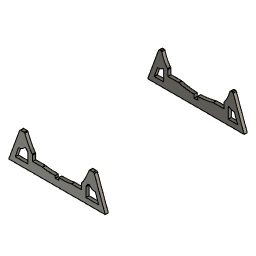
Revell Flower Class stand (Autodesk Fusion 360 design; units mm, degrees)
Autodesk Fusion 360 part; units mm, degrees
note: some values were not read from the file. Chosen so that the rebuilt part matches the saved one: which face or edge a step refers to.
ref_plane "WorkPlane1" through (0, -135, 0) normal (0, 1, 0) x (0, 0, 1) in component "Fore"
sketch "Sketch1" plane through (0, -135, 0) normal (0, 1, 0) x (1, 0, 0) in component "Fore"
  line L0 (0, 0) -> (0, -12.5)
  line L1 (0, -12.5) -> (-3.5, -12.5)
  line L2 (-3.5, -12.5) -> (-3.5, -17)
  spline S0 degree 5 poles (-3.5, -17) (-4.4939, -17) (-6.4799, -17.0057) (-9.4532, -17.0312) (-13.4085, -17.1077) (-18.3463, -17.343) (-22.2994, -17.7362) (-25.2695, -18.2105) (-27.2527, -18.6198) (-28.245, -18.8477) knots 0 0 0 0 0 0 0.2 0.4 0.6 0.8 1 1 1 1 1 1
  line L3 (-28.245, -18.8477) -> (-47.4725, -18.8477)
  line L4 (-47.4725, -18.8477) -> (-47.4725, -30.1587)
  spline S1 degree 5 poles (-47.4725, -30.1587) (-47.8872, -30.6443) (-48.7402, -31.6972) (-50.0906, -33.5222) (-52.0431, -36.4804) (-54.8605, -41.4812) (-57.606, -47.1812) (-60.0804, -52.8922) (-61.9442, -57.4399) (-62.9296, -59.899) knots 0 0 0 0 0 0 0.2 0.4 0.6 0.8 1 1 1 1 1 1
  line L5 (-62.9296, -59.899) -> (-72.0582, -59.899)
  line L6 (-72.0582, -59.899) -> (-93.742, 0)
  line L7 (-93.742, 0) -> (0, 0)
  line L8 (-60.4227, -53.6433) -> (-65.4365, -66.1546)
  line L9 (-0.969, -17) -> (-6.031, -17)
  line L10 (-25.7289, -18.2698) -> (-30.7611, -19.4256)
  line L11 (-74.7277, -28.7021) -> (-81.0107, -10.108)
  line L12 (-81.0107, -10.108) -> (-56.4844, -10.108)
  line L13 (-56.4844, -10.108) -> (-56.4844, -29.2553)
  line L14 (-56.4844, -29.2553) -> (-59.3576, -33.4494)
  spline S2 degree 5 poles (-59.3576, -33.4494) (-59.567, -33.755) (-60.0141, -34.2929) (-60.7709, -34.8796) (-61.8493, -35.2265) (-62.983, -34.9858) (-63.6467, -34.1638) (-64.3685, -32.9555) (-65.6314, -31.5945) (-67.452, -30.2924) (-69.7221, -29.2481) (-71.72, -28.7519) (-73.231, -28.6255) (-74.2302, -28.6572) (-74.7277, -28.7021) knots 0 0 0 0 0 0 0.1 0.2 0.3 0.4 0.5 0.6 0.7 0.8 0.9 1 1 1 1 1 1
  line L15 (-72.7235, -28.5213) -> (-76.7319, -28.8828)
  line L16 (-62.8657, -35.095) -> (-64.2557, -33.3052)
  line L17 (-57.9122, -31.3395) -> (-60.8031, -35.5592)
  point P0 (-63.5607, -34.2001)
  dimension "d2" = 12.5
  dimension "d3" = 4.5
  dimension "d4" = 3.5
  constraint coincident L0.start L7.end
  constraint vertical L0
  constraint perpendicular L0 L1
  constraint perpendicular L1 L2
  constraint horizontal L3
  constraint perpendicular L3 L4
  constraint horizontal L5
  constraint perpendicular L0 L7
  constraint midpoint S1.end L8
  constraint midpoint L2.end L9
  constraint horizontal L9
  constraint midpoint S0.end L10
  constraint horizontal L12
  constraint perpendicular L12 L13
  constraint midpoint L11.start L15
  constraint midpoint P0 L16
  constraint midpoint L14.end L17
  measures "d2" distance of L0.start L0.end
  measures "d3" distance of L1.end L2.end
  measures "d4" distance of L0.end L1.end
ref_plane "WorkPlane1" through (0, 135, 0) normal (0, 1, 0) x (0, 0, 1) in component "Aft"
sketch "Sketch1 (2)" plane through (0, 135, 0) normal (0, 1, 0) x (1, 0, 0) in component "Aft"
  line L0 (0, 0) -> (0, -12.5)
  line L1 (0, -12.5) -> (-3.5, -12.5)
  line L2 (-3.5, -12.5) -> (-3.5, -19)
  spline S0 degree 5 poles (-3.5, -19) (-4.3766, -19) (-6.2365, -19.0347) (-9.3458, -19.191) (-14.0327, -19.5941) (-20.4233, -20.4205) (-25.6959, -21.3969) (-29.6354, -22.3657) (-32.2417, -23.1312) (-33.54, -23.5438) knots 0 0 0 0 0 0 0.2 0.4 0.6 0.8 1 1 1 1 1 1
  line L3 (-33.54, -23.5438) -> (-54.6225, -23.5438)
  line L4 (-54.6225, -23.5438) -> (-54.6225, -35.6286)
  spline S1 degree 5 poles (-54.6225, -35.6286) (-55.2677, -36.2626) (-56.496, -37.575) (-58.1518, -39.6766) (-60.0494, -42.7526) (-62.1582, -47.2156) (-63.8351, -51.5517) (-65.178, -55.4393) (-66.1249, -58.3579) (-66.6112, -59.899) knots 0 0 0 0 0 0 0.2 0.4 0.6 0.8 1 1 1 1 1 1
  line L5 (-72.0582, -59.899) -> (-93.742, 0)
  line L6 (-72.0582, -59.899) -> (-66.6112, -59.899)
  line L7 (-65.3783, -55.9921) -> (-67.8442, -63.8058)
  line L8 (-53.0217, -34.0557) -> (-56.2233, -37.2015)
  line L9 (-93.742, 0) -> (0, 0)
  line L10 (-74.5428, -28.526) -> (-81.0107, -10.108)
  line L11 (-81.0107, -10.108) -> (-62.7924, -10.108)
  line L12 (-62.7924, -10.108) -> (-62.7924, -32.6534)
  spline S2 degree 5 poles (-62.7924, -32.6534) (-63.1413, -32.3681) (-63.8532, -31.8115) (-64.9633, -31.0185) (-66.5337, -30.0508) (-68.7209, -29.0636) (-70.7629, -28.564) (-72.5414, -28.4344) (-73.8545, -28.4744) (-74.5428, -28.526) knots 0 0 0 0 0 0 0.2 0.4 0.6 0.8 1 1 1 1 1 1
  line L13 (-72.8582, -28.3997) -> (-76.2275, -28.6524)
  line L14 (-1.2608, -19) -> (-5.7392, -19)
  line L15 (-30.2257, -22.4904) -> (-36.8542, -24.5973)
  point P0 (-81.0107, -10.108)
  dimension "d16" = 12.5
  dimension "d17" = 3.5
  dimension "d18" = 6.5
  constraint coincident L0.start L9.end
  constraint vertical L0
  constraint perpendicular L0 L1
  constraint perpendicular L1 L2
  constraint horizontal L3
  constraint perpendicular L3 L4
  constraint coincident L5.start L6.start
  constraint horizontal L6
  constraint coincident S1.end L6.end
  constraint midpoint S1.end L7
  constraint midpoint L4.end L8
  constraint coincident L5.end L9.start
  constraint coincident P0 L10.end
  constraint horizontal L11
  constraint perpendicular L11 L12
  constraint midpoint L10.start L13
  constraint midpoint L2.end L14
  constraint horizontal L14
  constraint midpoint S0.end L15
  measures "d16" distance of L0.start L0.end
  measures "d17" distance of L0.end L1.end
  measures "d18" distance of L1.end L2.end
extrude "Extrude2" add sketch "Sketch1" along normal mid plane 6 makes body 1 in component "Fore"
fillet "Fillet6" radius 2 3 edges at (-28.245, -135, 18.8477) (-47.4725, -135, 30.1587) (-72.0582, -135, 59.899) on bodies 1 in component "Fore"
fillet "Fillet7" radius 1.5 1 edges at (-62.9296, -135, 59.899) on bodies 1 in component "Fore"
fillet "Fillet8" radius 1 1 edges at (-74.7277, -135, 28.7021) on bodies 1 in component "Fore"
fillet "Fillet9" radius 3.5 1 edges at (-56.4844, -135, 29.2553) on bodies 1 in component "Fore"
extrude "Extrude1" add sketch "Sketch1 (2)" along normal mid plane 6 separate body makes body 2 in component "Aft"
fillet "Fillet1" radius 2 3 edges at (-33.54, 135, 23.5438) (-54.6225, 135, 35.6286) (-72.0582, 135, 59.899) on bodies 2 in component "Aft"
fillet "Fillet2" radius 1.5 2 edges at (-66.6112, 136.5, 59.899) (-66.6112, 133.5, 59.899) on bodies 2 in component "Aft"
fillet "Fillet3" radius 1 1 edges at (-74.5428, 135, 28.526) on bodies 2 in component "Aft"
fillet "Fillet4" radius 0.7 2 edges at (-62.7924, 136.5, 32.6534) (-62.7924, 133.5, 32.6534) on bodies 2 in component "Aft"
mirror "Mirror2" about plane through (0, 0, 0) normal (1, 0, 0) of bodies 1 makes body 3 in component "Fore"
combine "Combine2" operation add target body 1 tool bodies 3 in component "Fore"
mirror "Mirror1" about plane through (0, 0, 0) normal (1, 0, 0) of bodies 2 makes body 4 in component "Aft"
combine "Combine1" operation add target body 2 tool bodies 4 in component "Aft"
component "Fore" placed x (1, 0, 0) y (0, 1, 0) z (0, 0, 1) at (0, 0, 0)
component "Aft" placed x (1, 0, 0) y (0, 1, 0) z (0, 0, 1) at (0, 0, 0)
equation "tolerance = 0 mm"
equation "materialThickness = 6 mm"
equation "d19 = materialThickness"
equation "d25 = materialThickness"
named bodies: "Body1"
